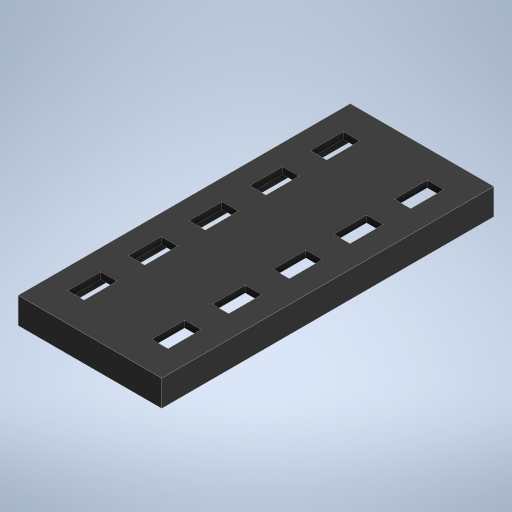
# Autodesk Inventor part: RelayCaseTop
Saved by Autodesk Inventor 2024 (Build 280153000, 153)
## iProperties
Created: 2023-08-11
Part Number: RelayCaseTop
Material: Rubber, Silicone
Document SubType Name: Modeling
Designer: 18179
Density: 1.25 g/cm^3
Appearance: Rubber - Black
Autodesk Inventor part; units mm, degrees
ref_plane "YZ Plane" through (0, 0, 0) normal (1, 0, 0) x (0, 1, 0)
ref_plane "XZ Plane" through (0, 0, 0) normal (0, 1, 0) x (-1, 0, 0)
ref_plane "XY Plane" through (0, 0, 0) normal (0, 0, 1) x (1, 0, 0)
sketch "Sketch4" plane through (0, 0, 0) normal (0, 1, 0) x (-1, 0, 0)
  line L0 (0, 0) -> (59.7662, 0)
  line L1 (59.7662, 0) -> (59.7662, -146.1262)
  line L2 (59.7662, -146.1262) -> (0, -146.1262)
  line L3 (0, -146.1262) -> (0, 0)
  line L4 (59.7662, 0) -> (53.4924, 0)
  line L5 (53.4924, 0) -> (53.4924, -9.5758)
  line L6 (53.4924, -9.5758) -> (59.7662, -9.5758)
  line L7 (59.7662, -9.5758) -> (59.7662, 0)
  line L8 (53.4924, -9.5758) -> (45.8724, -9.5758)
  line L9 (45.8724, -9.5758) -> (45.8724, -24.8158)
  line L10 (45.8724, -24.8158) -> (53.4924, -24.8158)
  line L11 (53.4924, -24.8158) -> (53.4924, -9.5758)
  line L12 (45.8724, -24.8158) -> (45.8724, -37.5158)
  line L13 (45.8724, -37.5158) -> (53.4924, -37.5158)
  line L14 (53.4924, -37.5158) -> (53.4924, -52.7558)
  line L15 (53.4924, -52.7558) -> (45.8724, -52.7558)
  line L16 (45.8724, -52.7558) -> (45.8724, -37.5158)
  line L17 (45.8724, -52.7558) -> (45.8724, -65.4558)
  line L18 (45.8724, -65.4558) -> (53.4924, -65.4558)
  line L19 (53.4924, -65.4558) -> (53.4924, -80.6958)
  line L20 (53.4924, -80.6958) -> (45.8724, -80.6958)
  line L21 (45.8724, -80.6958) -> (45.8724, -65.4558)
  line L22 (45.8724, -80.6958) -> (45.8724, -93.3958)
  line L23 (45.8724, -93.3958) -> (53.4924, -93.3958)
  line L24 (53.4924, -93.3958) -> (53.4924, -108.6358)
  line L25 (53.4924, -108.6358) -> (45.8724, -108.6358)
  line L26 (45.8724, -108.6358) -> (45.8724, -93.3958)
  line L27 (45.8724, -108.6358) -> (45.8724, -121.3358)
  line L28 (45.8724, -121.3358) -> (53.4924, -121.3358)
  line L29 (53.4924, -121.3358) -> (53.4924, -136.5758)
  line L30 (53.4924, -136.5758) -> (45.8724, -136.5758)
  line L31 (45.8724, -136.5758) -> (45.8724, -121.3358)
  line L32 (0, 0) -> (7.1628, 0)
  line L33 (7.1628, 0) -> (7.1628, -9.5758)
  line L34 (7.1628, -9.5758) -> (0, -9.5758)
  line L35 (0, -9.5758) -> (0, 0)
  line L36 (53.4924, -9.5758) -> (7.1628, -9.5758)
  line L37 (30.3276, -9.5758) -> (30.3276, -4.7879)
  line L38 (7.1628, -9.5758) -> (14.7828, -9.5758)
  line L39 (14.7828, -9.5758) -> (14.7828, -24.8158)
  line L40 (14.7828, -24.8158) -> (7.1628, -24.8158)
  line L41 (7.1628, -24.8158) -> (7.1628, -9.5758)
  line L42 (14.7828, -37.5158) -> (7.1628, -37.5158)
  line L43 (7.1628, -37.5158) -> (7.1628, -52.7558)
  line L44 (7.1628, -52.7558) -> (14.7828, -52.7558)
  line L45 (14.7828, -52.7558) -> (14.7828, -37.5158)
  line L46 (14.7828, -65.4558) -> (7.1628, -65.4558)
  line L47 (7.1628, -65.4558) -> (7.1628, -80.6958)
  line L48 (7.1628, -80.6958) -> (14.7828, -80.6958)
  line L49 (14.7828, -80.6958) -> (14.7828, -65.4558)
  line L50 (14.7828, -93.3958) -> (7.1628, -93.3958)
  line L51 (7.1628, -93.3958) -> (7.1628, -108.6358)
  line L52 (7.1628, -108.6358) -> (14.7828, -108.6358)
  line L53 (14.7828, -108.6358) -> (14.7828, -93.3958)
  line L54 (14.7828, -121.3358) -> (7.1628, -121.3358)
  line L55 (7.1628, -121.3358) -> (7.1628, -136.5758)
  line L56 (7.1628, -136.5758) -> (14.7828, -136.5758)
  line L57 (14.7828, -136.5758) -> (14.7828, -121.3358)
  line L58 (7.1628, -9.5758) -> (53.4924, -9.5758)
  line L59 (0, 0) -> (0, -146.1262)
  line L60 (0, -146.1262) -> (59.7662, -146.1262)
  line L61 (59.7662, -146.1262) -> (59.7662, 0)
  line L62 (62.9412, 0) -> (62.9412, -149.3012)
  line L63 (62.9412, -149.3012) -> (-3.175, -149.3012)
  line L64 (-3.175, -149.3012) -> (-3.175, 0)
  line L65 (0, 0.508) -> (59.7662, 0.508)
  line L66 (0, 3.683) -> (59.7662, 3.683)
  line L67 (62.9412, 0) -> (59.7662, 0)
  line L68 (59.7662, 0) -> (59.7662, 3.683)
  line L69 (59.7662, 3.683) -> (62.9412, 3.683)
  line L70 (62.9412, 3.683) -> (62.9412, 0)
  line L71 (-3.175, 0) -> (0, 0)
  line L72 (0, 0) -> (0, 3.683)
  line L73 (0, 3.683) -> (-3.175, 3.683)
  line L74 (-3.175, 3.683) -> (-3.175, 0)
  line L75 (0, 0.508) -> (0, 0.508)
  line L76 (0, 0.508) -> (0, 0)
  line L77 (0, 0) -> (0, 0)
  line L78 (0, 0) -> (0, 0.508)
  line L79 (59.7662, 0.508) -> (59.7662, 0.508)
  line L80 (59.7662, 0.508) -> (59.7662, 0)
  line L81 (59.7662, 0) -> (59.7662, 0)
  line L82 (59.7662, 0) -> (59.7662, 0.508)
  point P0 (59.7662, 0)
  dimension "d503" = 59.7662
  dimension "d504" = 146.1262
  dimension "d505" = 6.2738
  dimension "d506" = 9.5758
  dimension "d507" = 7.62
  dimension "d508" = 15.24
  dimension "d509" = 12.7
  dimension "d510" = 7.62
  dimension "d511" = 15.24
  dimension "d512" = 12.7
  dimension "d513" = 7.62
  dimension "d514" = 15.24
  dimension "d515" = 12.7
  dimension "d516" = 7.62
  dimension "d517" = 15.24
  dimension "d518" = 12.7
  dimension "d519" = 7.62
  dimension "d520" = 15.24
  dimension "d521" = 7.1628
  dimension "d522" = 9.5758
  dimension "d529" = 3.175
  dimension "d530" = 0.508
  dimension "d531" = 3.175
  constraints: 166 end point, 28 equal length, 21 symmetric about line, 12 horizontal, 12 perpendicular, 5 vertical, 1 collinear, 1 midpoint, 4 other
  measures "d503" distance of L1.end L2.end
  measures "d504" distance of L0.end L1.end
  measures "d505" distance of L6.end L5.end
  measures "d506" distance of L5.end L4.end
  measures "d507" distance of L10.end L9.end
  measures "d508" distance of L9.end L8.end
  measures "d509" distance of L9.end L12.end
  measures "d510" distance of L14.end L15.end
  measures "d511" distance of L13.end L14.end
  measures "d512" distance of L15.end L17.end
  measures "d513" distance of L19.end L20.end
  measures "d514" distance of L18.end L19.end
  measures "d515" distance of L20.end L22.end
  measures "d516" distance of L24.end L25.end
  measures "d517" distance of L23.end L24.end
  measures "d518" distance of L25.end L27.end
  measures "d519" distance of L29.end L30.end
  measures "d520" distance of L28.end L29.end
  measures "d521" distance of L33.end L34.end
  measures "d522" distance of L32.end L33.end
  measures "d529" distance between parallel lines of L60 L63
  measures "d530" distance between parallel lines of L0 L65
  measures "d531" distance between parallel lines of L65 L66
extrude "Extrusion4" add sketch "Sketch4" along normal blind 3.175 contours L72 L65 L68 L0 | L0 L33 L34 L3 | L3 L2 L1 L67 L62 L63 L64 L71 | L71 L74 L73 L72 | L0 L5 L8 L36 L33 | L34 L41 L40 L39 L36 L9 L10 L11 L6 L1 L2 L3 | L72 L66 L68 L65 | L0 L1 L6 L5 | L68 L69 L70 L67
sketch "Sketch5" plane through (0, 0, 0) normal (0, -1, 0) x (1, 0, 0)
  line L0 (-7.1628, -9.5758) -> (-14.7828, -9.5758) projected
  line L1 (-7.1628, -24.8158) -> (-7.1628, -9.5758) projected
  line L2 (-14.7828, -24.8158) -> (-7.1628, -24.8158) projected
  line L3 (-14.7828, -9.5758) -> (-14.7828, -24.8158) projected
  line L4 (-53.4924, -9.5758) -> (-53.4924, -24.8158) projected
  line L5 (-45.8724, -9.5758) -> (-53.4924, -9.5758) projected
  line L6 (-45.8724, -24.8158) -> (-45.8724, -9.5758) projected
  line L7 (-53.4924, -24.8158) -> (-45.8724, -24.8158) projected
  line L8 (-45.8724, -121.3358) -> (-53.4924, -121.3358) projected
  line L9 (-45.8724, -136.5758) -> (-45.8724, -121.3358) projected
  line L10 (-53.4924, -136.5758) -> (-45.8724, -136.5758) projected
  line L11 (-53.4924, -121.3358) -> (-53.4924, -136.5758) projected
  line L12 (-45.8724, -108.6358) -> (-45.8724, -93.3958) projected
  line L13 (-53.4924, -108.6358) -> (-45.8724, -108.6358) projected
  line L14 (-53.4924, -93.3958) -> (-53.4924, -108.6358) projected
  line L15 (-45.8724, -93.3958) -> (-53.4924, -93.3958) projected
  line L16 (-45.8724, -80.6958) -> (-45.8724, -65.4558) projected
  line L17 (-53.4924, -80.6958) -> (-45.8724, -80.6958) projected
  line L18 (-53.4924, -65.4558) -> (-53.4924, -80.6958) projected
  line L19 (-45.8724, -65.4558) -> (-53.4924, -65.4558) projected
  line L20 (-45.8724, -52.7558) -> (-45.8724, -37.5158) projected
  line L21 (-53.4924, -52.7558) -> (-45.8724, -52.7558) projected
  line L22 (-53.4924, -37.5158) -> (-53.4924, -52.7558) projected
  line L23 (-45.8724, -37.5158) -> (-53.4924, -37.5158) projected
  line L24 (-7.1628, -80.6958) -> (-7.1628, -65.4558) projected
  line L25 (-14.7828, -80.6958) -> (-7.1628, -80.6958) projected
  line L26 (-14.7828, -65.4558) -> (-14.7828, -80.6958) projected
  line L27 (-7.1628, -65.4558) -> (-14.7828, -65.4558) projected
  line L28 (-14.7828, -121.3358) -> (-14.7828, -136.5758) projected
  line L29 (-7.1628, -121.3358) -> (-14.7828, -121.3358) projected
  line L30 (-7.1628, -136.5758) -> (-7.1628, -121.3358) projected
  line L31 (-14.7828, -136.5758) -> (-7.1628, -136.5758) projected
  line L32 (-14.7828, -37.5158) -> (-14.7828, -52.7558) projected
  line L33 (-7.1628, -37.5158) -> (-14.7828, -37.5158) projected
  line L34 (-7.1628, -52.7558) -> (-7.1628, -37.5158) projected
  line L35 (-14.7828, -52.7558) -> (-7.1628, -52.7558) projected
  line L36 (-7.1628, -108.6358) -> (-7.1628, -93.3958) projected
  line L37 (-14.7828, -108.6358) -> (-7.1628, -108.6358) projected
  line L38 (-14.7828, -93.3958) -> (-14.7828, -108.6358) projected
  line L39 (-7.1628, -93.3958) -> (-14.7828, -93.3958) projected
  line L40 (-3.048, -3.048) -> (-3.048, -143.0782)
  line L41 (-3.048, -143.0782) -> (-56.7182, -143.0782)
  line L42 (-56.7182, -143.0782) -> (-56.7182, -3.048)
  line L43 (-56.7182, -3.048) -> (-3.048, -3.048)
  line L44 (-62.9412, 3.683) -> (3.175, 3.683) projected
  line L45 (3.175, 3.683) -> (3.175, -149.3012) projected
  line L46 (3.175, -149.3012) -> (-62.9412, -149.3012) projected
  line L47 (-62.9412, -149.3012) -> (-62.9412, 3.683) projected
  line L48 (0, 0.508) -> (-59.7662, 0.508)
  line L49 (-59.7662, 0.508) -> (-59.7662, -146.1262)
  line L50 (-59.7662, -146.1262) -> (0, -146.1262)
  line L51 (0, -146.1262) -> (0, 0.508)
  point P0 (0, 0)
  dimension "d532" = 3.175
  constraints: 16 end point, 3 other
  measures "d532" distance between parallel lines of L44 L48
extrude "Extrusion5" add sketch "Sketch5" along normal blind 8.89 contours L44 L45 L46 L47
body "Solid2"
